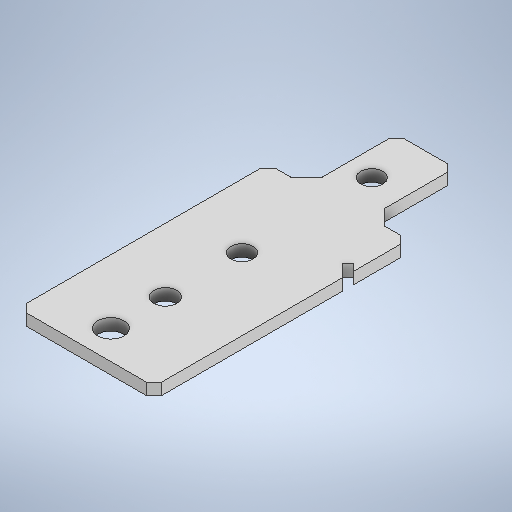
# Autodesk Inventor part: B3-camera
Saved by Autodesk Inventor 2025.2 (Build 292293000, 293)
## iProperties
Created: 2025-11-05
Part Number: B3-camera
Material: 일반
Document SubType Name: Modeling
Designer: RunGeun
Density: 1 g/cm^3
Appearance: 기본값
Author: RunGeun
Autodesk Inventor part; units mm, degrees
ref_plane "YZ Plane" through (0, 0, 0) normal (1, 0, 0) x (0, 1, 0)
ref_plane "XZ Plane" through (0, 0, 0) normal (0, 1, 0) x (-1, 0, 0)
ref_plane "XY Plane" through (0, 0, 0) normal (0, 0, 1) x (1, 0, 0)
sketch "스케치1" plane through (0, 0, 0) normal (0, 1, 0) x (-1, 0, 0)
  line L0 (2, 0) -> (32.9, 0)
  line L1 (34.9, -2) -> (34.9, -62.2175)
  line L2 (23, -87.35) -> (12, -87.35)
  circle A0 centre (18.5, -7.4) radius 3.4
  circle A1 centre (18.5, -21.4) radius 2.95
  line L3 (25, -87.35) -> (10, -87.35)
  line L4 (10, -85.35) -> (10, -65.3675)
  line L5 (25, -64.2175) -> (25, -85.35)
  line L6 (29, -64.2175) -> (32.9, -64.2175)
  line L7 (25, -69.1747) -> (25, -68.2175)
  line L8 (6, -65.3675) -> (2, -65.3675)
  line L9 (10, -72.4067) -> (10, -69.3675)
  line L10 (34.9, -2) -> (32.9, 0)
  line L11 (2, 0) -> (0, -2)
  line L12 (10, -85.35) -> (12, -87.35)
  line L13 (23, -87.35) -> (25, -85.35)
  line L14 (32.9, -64.2175) -> (34.9, -62.2175)
  line L15 (2, -65.3675) -> (0, -63.3675)
  line L16 (25, -68.2175) -> (29, -64.2175)
  line L17 (10, -69.3675) -> (6, -65.3675)
  circle A2 centre (18.5, -41.1) radius 2.85
  circle A3 centre (18.5, -74.5) radius 2.85
  line L18 (0, -51.2702) -> (1.7469, -53.0172)
  line L19 (1.7469, -53.0172) -> (3.1319, -51.6322)
  line L20 (3.1319, -51.6322) -> (0, -48.5004)
  line L21 (0, -63.3675) -> (0, -51.2702)
  line L22 (0, -48.5004) -> (0, -2)
  point P0 (0, 0)
  point P1 (34.9, 0)
  point P2 (0, -65.3675)
  point P3 (34.9, -64.2175)
  point P4 (17.5, -87.35)
  point P5 (25, -68.2175)
  dimension "d0" = 13
  dimension "d2" = 4
  dimension "d3" = 6.8
  dimension "d4" = 5.9
  dimension "d8" = 63
  dimension "d13" = 2
  dimension "d14" = 2
  dimension "d15" = 2
  dimension "d16" = 2
  dimension "d17" = 2
  dimension "d18" = 2
  dimension "d19" = 2
  dimension "d20" = 2
  dimension "d21" = 2
  dimension "d22" = 2
  dimension "d23" = 2
  dimension "d24" = 2
  dimension "d25" = 4
  dimension "d26" = 4
  dimension "d27" = 4
  dimension "d28" = 4
  dimension "d29" = 5.7
  dimension "d30" = 5.7
  dimension "d38" = 14
  dimension "d39" = 19.7
  dimension "d40" = 33.4
  constraints: 46 end point, 14 point on line, 5 parallel, 4 centre point, 4 horizontal, 2 perpendicular, 1 midpoint
  measures "d0" distance edge to line of A0 L1
  measures "d2" distance edge to line of A0 L0
  measures "d3" diameter of A0
  measures "d4" diameter of A1
  measures "d8" distance edge to line of A1 L2
  measures "d13" distance of L1.start point (34.9, 0)
  measures "d14" distance of L0.end point (34.9, 0)
  measures "d15" distance of L0.start point (0, 0)
  measures "d16" distance of L11.end point (0, 0)
  measures "d17" distance of L4.start L3.end
  measures "d18" distance of L2.end L3.end
  measures "d19" distance of L2.start L3.start
  measures "d20" distance of L5.end L3.start
  measures "d21" distance of L6.end point (34.9, -64.217)
  measures "d22" distance of L1.end point (34.9, -64.217)
  measures "d23" distance of L8.end point (0, -65.367)
  measures "d24" distance of L15.end point (0, -65.367)
  measures "d25" distance of L7.end L5.start
  measures "d26" distance of L6.start L5.start
  measures "d27" distance of L9.end L4.end
  measures "d28" distance of L8.start L4.end
  measures "d29" diameter of A2
  measures "d30" diameter of A3
  measures "d38" distance of A1.centre A0.centre
  measures "d39" distance of A2.centre A1.centre
  measures "d40" distance of A3.centre A2.centre
extrude "돌출2" add sketch "스케치1" along normal blind 3
equation "\"d14\" = d13"
equation "\"d15\" = d13"
equation "\"d16\" = d15"
equation "\"d17\" = d13"
equation "\"d18\" = d17"
equation "\"d19\" = d13"
equation "\"d20\" = d19"
equation "\"d21\" = d13"
equation "\"d22\" = d21"
equation "\"d23\" = d13"
equation "\"d24\" = d23"
equation "\"d26\" = d25"
equation "\"d27\" = d25"
equation "\"d28\" = d27"
equation "\"d30\" = d29"
equation "\"d33\" = d32"
equation "\"d32\" = 18.5"
